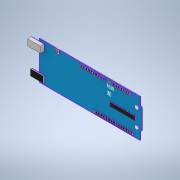
# Autodesk Inventor part: Arduino board
Saved by Autodesk Inventor 2021 (Build 250183000, 183)
## iProperties
Created: 2021-06-29
Part Number: Arduino board
Material: Generic
Document SubType Name: Modeling
Designer: shifa
Density: 1 g/cm^3
Appearance: Default
Author: shifa
Autodesk Inventor part; units mm, degrees
ref_plane "YZ Plane" through (0, 0, 0) normal (1, 0, 0) x (0, 1, 0)
ref_plane "XZ Plane" through (0, 0, 0) normal (0, 1, 0) x (-1, 0, 0)
ref_plane "XY Plane" through (0, 0, 0) normal (0, 0, 1) x (1, 0, 0)
sketch "Sketch1" plane through (0, 0, 0) normal (0, 0, 1) x (1, 0, 0)
  line L0 (-70, -14.9942) -> (-70, 15.0058)
  line L1 (-70, 15.0058) -> (10, 15.0058)
  line L2 (10, 15.0058) -> (10, 9)
  line L3 (10, 9) -> (11.2892, 8.1067)
  line L4 (11.2892, 8.1067) -> (11.2892, -7.6953)
  line L5 (11.2892, -7.6953) -> (10, -8.7379)
  line L6 (10, -8.7379) -> (10, -14.9942)
  line L7 (10, -14.9942) -> (-70, -14.9942)
  line L8 (-56.9712, 15.0058) -> (-53.9712, 15.0058)
  line L9 (-53.9712, 15.0058) -> (-53.9712, 12.0058)
  line L10 (-53.9712, 12.0058) -> (-56.9712, 12.0058)
  line L11 (-56.9712, 12.0058) -> (-56.9712, 15.0058)
  circle A0 centre (-55.5993, 13.6025) radius 1
  line L12 (-76.1027, 13.1862) -> (-66.1027, 13.1862)
  line L13 (-66.1027, 13.1862) -> (-66.1027, 8.1862)
  line L14 (-66.1027, 8.1862) -> (-76.1027, 8.1862)
  line L15 (-76.1027, 8.1862) -> (-76.1027, 13.1862)
  line L16 (-13.5947, -0.1189) -> (6.4053, -0.1189)
  line L17 (6.4053, -0.1189) -> (6.4053, -3.1189)
  line L18 (6.4053, -3.1189) -> (-13.5947, -3.1189)
  line L19 (-13.5947, -3.1189) -> (-13.5947, -0.1189)
  line L20 (-75.8788, -8.319) -> (-65.8788, -8.319)
  line L21 (-65.8788, -8.319) -> (-65.8788, -13.319)
  line L22 (-65.8788, -13.319) -> (-75.8788, -13.319)
  line L23 (-75.8788, -13.319) -> (-75.8788, -8.319)
  circle A1 centre (7.656, 6.6067) radius 1.5
  circle A2 centre (7.656, -7.1392) radius 1.5
  line L24 (2.5046, 14.0058) -> (2.5046, 12.0058)
  line L25 (2.5046, 12.0058) -> (-14.4954, 12.0058)
  line L26 (-14.4954, 14.0058) -> (2.5046, 14.0058)
  line L27 (-14.4954, 12.0058) -> (-14.4954, 14.0058)
  line L28 (-17.3599, 14.0058) -> (-17.3599, 12.0058)
  line L29 (-17.3599, 12.0058) -> (-37.8599, 12.0058)
  line L30 (-37.8599, 14.0058) -> (-17.3599, 14.0058)
  line L31 (-37.8599, 12.0058) -> (-37.8599, 14.0058)
  line L32 (-14.4954, 14.0058) -> (2.5046, 14.0058)
  line L33 (-14.4954, 12.0058) -> (-14.4954, 14.0058)
  line L34 (2.5046, 12.0058) -> (-14.4954, 12.0058)
  line L35 (2.5046, 14.0058) -> (2.5046, 12.0058)
  line L36 (-8.0961, -12.0647) -> (4.4039, -12.0647)
  line L37 (-8.0961, -14.0647) -> (-8.0961, -12.0647)
  line L38 (4.4039, -14.0647) -> (-8.0961, -14.0647)
  line L39 (4.4039, -12.0647) -> (4.4039, -14.0647)
  line L40 (-26.6201, -12.0647) -> (-9.6201, -12.0647)
  line L41 (-26.6201, -14.0647) -> (-26.6201, -12.0647)
  line L42 (-9.6201, -14.0647) -> (-26.6201, -14.0647)
  line L43 (-9.6201, -12.0647) -> (-9.6201, -14.0647)
  line L44 (-37.2773, 13.7542) -> (-35.7773, 13.7542)
  line L45 (-35.7773, 13.7542) -> (-35.7773, 12.2542)
  line L46 (-35.7773, 12.2542) -> (-37.2773, 12.2542)
  line L47 (-37.2773, 12.2542) -> (-37.2773, 13.7542)
  line L48 (-35.2773, 13.7542) -> (-33.7773, 13.7542)
  line L49 (-35.2773, 12.2542) -> (-35.2773, 13.7542)
  line L50 (-33.7773, 12.2542) -> (-35.2773, 12.2542)
  line L51 (-33.7773, 13.7542) -> (-33.7773, 12.2542)
  line L52 (-33.2773, 13.7542) -> (-31.7773, 13.7542)
  line L53 (-33.2773, 12.2542) -> (-33.2773, 13.7542)
  line L54 (-31.7773, 12.2542) -> (-33.2773, 12.2542)
  line L55 (-31.7773, 13.7542) -> (-31.7773, 12.2542)
  line L56 (-31.2773, 13.7542) -> (-29.7773, 13.7542)
  line L57 (-31.2773, 12.2542) -> (-31.2773, 13.7542)
  line L58 (-29.7773, 12.2542) -> (-31.2773, 12.2542)
  line L59 (-29.7773, 13.7542) -> (-29.7773, 12.2542)
  line L60 (-29.2773, 13.7542) -> (-27.7773, 13.7542)
  line L61 (-29.2773, 12.2542) -> (-29.2773, 13.7542)
  line L62 (-27.7773, 12.2542) -> (-29.2773, 12.2542)
  line L63 (-27.7773, 13.7542) -> (-27.7773, 12.2542)
  line L64 (-27.2773, 13.7542) -> (-25.7773, 13.7542)
  line L65 (-27.2773, 12.2542) -> (-27.2773, 13.7542)
  line L66 (-25.7773, 12.2542) -> (-27.2773, 12.2542)
  line L67 (-25.7773, 13.7542) -> (-25.7773, 12.2542)
  line L68 (-25.2773, 13.7542) -> (-23.7773, 13.7542)
  line L69 (-25.2773, 12.2542) -> (-25.2773, 13.7542)
  line L70 (-23.7773, 12.2542) -> (-25.2773, 12.2542)
  line L71 (-23.7773, 13.7542) -> (-23.7773, 12.2542)
  line L72 (-23.2773, 13.7542) -> (-21.7773, 13.7542)
  line L73 (-23.2773, 12.2542) -> (-23.2773, 13.7542)
  line L74 (-21.7773, 12.2542) -> (-23.2773, 12.2542)
  line L75 (-21.7773, 13.7542) -> (-21.7773, 12.2542)
  line L76 (-21.2773, 13.7542) -> (-19.7773, 13.7542)
  line L77 (-21.2773, 12.2542) -> (-21.2773, 13.7542)
  line L78 (-19.7773, 12.2542) -> (-21.2773, 12.2542)
  line L79 (-19.7773, 13.7542) -> (-19.7773, 12.2542)
  line L80 (-19.2773, 13.7542) -> (-17.7773, 13.7542)
  line L81 (-19.2773, 12.2542) -> (-19.2773, 13.7542)
  line L82 (-17.7773, 12.2542) -> (-19.2773, 12.2542)
  line L83 (-17.7773, 13.7542) -> (-17.7773, 12.2542)
  line L84 (-25.4265, -12.3263) -> (-23.9265, -12.3263)
  line L85 (-23.9265, -12.3263) -> (-23.9265, -13.8263)
  line L86 (-23.9265, -13.8263) -> (-25.4265, -13.8263)
  line L87 (-25.4265, -13.8263) -> (-25.4265, -12.3263)
  line L88 (-13.5947, 13.7542) -> (-12.0947, 13.7542)
  line L89 (-12.0947, 13.7542) -> (-12.0947, 12.2542)
  line L90 (-12.0947, 12.2542) -> (-13.5947, 12.2542)
  line L91 (-13.5947, 12.2542) -> (-13.5947, 13.7542)
  line L92 (-7.6221, -12.359) -> (-6.1221, -12.359)
  line L93 (-6.1221, -12.359) -> (-6.1221, -13.859)
  line L94 (-6.1221, -13.859) -> (-7.6221, -13.859)
  line L95 (-7.6221, -13.859) -> (-7.6221, -12.359)
  line L96 (-11.5947, 13.7542) -> (-10.0947, 13.7542)
  line L97 (-11.5947, 12.2542) -> (-11.5947, 13.7542)
  line L98 (-10.0947, 13.7542) -> (-10.0947, 12.2542)
  line L99 (-10.0947, 12.2542) -> (-11.5947, 12.2542)
  line L100 (-9.5947, 13.7542) -> (-8.0947, 13.7542)
  line L101 (-9.5947, 12.2542) -> (-9.5947, 13.7542)
  line L102 (-8.0947, 13.7542) -> (-8.0947, 12.2542)
  line L103 (-8.0947, 12.2542) -> (-9.5947, 12.2542)
  line L104 (-7.5947, 13.7542) -> (-6.0947, 13.7542)
  line L105 (-7.5947, 12.2542) -> (-7.5947, 13.7542)
  line L106 (-6.0947, 13.7542) -> (-6.0947, 12.2542)
  line L107 (-6.0947, 12.2542) -> (-7.5947, 12.2542)
  line L108 (-5.5947, 13.7542) -> (-4.0947, 13.7542)
  line L109 (-5.5947, 12.2542) -> (-5.5947, 13.7542)
  line L110 (-4.0947, 13.7542) -> (-4.0947, 12.2542)
  line L111 (-4.0947, 12.2542) -> (-5.5947, 12.2542)
  line L112 (-3.5947, 13.7542) -> (-2.0947, 13.7542)
  line L113 (-3.5947, 12.2542) -> (-3.5947, 13.7542)
  line L114 (-2.0947, 13.7542) -> (-2.0947, 12.2542)
  line L115 (-2.0947, 12.2542) -> (-3.5947, 12.2542)
  line L116 (-1.5947, 13.7542) -> (-0.0947, 13.7542)
  line L117 (-1.5947, 12.2542) -> (-1.5947, 13.7542)
  line L118 (-0.0947, 13.7542) -> (-0.0947, 12.2542)
  line L119 (-0.0947, 12.2542) -> (-1.5947, 12.2542)
  line L120 (0.4053, 13.7542) -> (1.9053, 13.7542)
  line L121 (0.4053, 12.2542) -> (0.4053, 13.7542)
  line L122 (1.9053, 13.7542) -> (1.9053, 12.2542)
  line L123 (1.9053, 12.2542) -> (0.4053, 12.2542)
  line L124 (-23.4265, -12.3263) -> (-21.9265, -12.3263)
  line L125 (-23.4265, -13.8263) -> (-23.4265, -12.3263)
  line L126 (-21.9265, -12.3263) -> (-21.9265, -13.8263)
  line L127 (-21.9265, -13.8263) -> (-23.4265, -13.8263)
  line L128 (-21.4265, -12.3263) -> (-19.9265, -12.3263)
  line L129 (-21.4265, -13.8263) -> (-21.4265, -12.3263)
  line L130 (-19.9265, -12.3263) -> (-19.9265, -13.8263)
  line L131 (-19.9265, -13.8263) -> (-21.4265, -13.8263)
  line L132 (-19.4265, -12.3263) -> (-17.9265, -12.3263)
  line L133 (-19.4265, -13.8263) -> (-19.4265, -12.3263)
  line L134 (-17.9265, -12.3263) -> (-17.9265, -13.8263)
  line L135 (-17.9265, -13.8263) -> (-19.4265, -13.8263)
  line L136 (-17.4265, -12.3263) -> (-15.9265, -12.3263)
  line L137 (-17.4265, -13.8263) -> (-17.4265, -12.3263)
  line L138 (-15.9265, -12.3263) -> (-15.9265, -13.8263)
  line L139 (-15.9265, -13.8263) -> (-17.4265, -13.8263)
  line L140 (-15.4265, -12.3263) -> (-13.9265, -12.3263)
  line L141 (-15.4265, -13.8263) -> (-15.4265, -12.3263)
  line L142 (-13.9265, -12.3263) -> (-13.9265, -13.8263)
  line L143 (-13.9265, -13.8263) -> (-15.4265, -13.8263)
  line L144 (-13.4265, -12.3263) -> (-11.9265, -12.3263)
  line L145 (-13.4265, -13.8263) -> (-13.4265, -12.3263)
  line L146 (-11.9265, -12.3263) -> (-11.9265, -13.8263)
  line L147 (-11.9265, -13.8263) -> (-13.4265, -13.8263)
  line L148 (-11.4265, -12.3263) -> (-9.9265, -12.3263)
  line L149 (-11.4265, -13.8263) -> (-11.4265, -12.3263)
  line L150 (-9.9265, -12.3263) -> (-9.9265, -13.8263)
  line L151 (-9.9265, -13.8263) -> (-11.4265, -13.8263)
  line L152 (-5.6221, -12.359) -> (-4.1221, -12.359)
  line L153 (-5.6221, -13.859) -> (-5.6221, -12.359)
  line L154 (-4.1221, -12.359) -> (-4.1221, -13.859)
  line L155 (-4.1221, -13.859) -> (-5.6221, -13.859)
  line L156 (-3.6221, -12.359) -> (-2.1221, -12.359)
  line L157 (-3.6221, -13.859) -> (-3.6221, -12.359)
  line L158 (-2.1221, -12.359) -> (-2.1221, -13.859)
  line L159 (-2.1221, -13.859) -> (-3.6221, -13.859)
  line L160 (-1.6221, -12.359) -> (-0.1221, -12.359)
  line L161 (-1.6221, -13.859) -> (-1.6221, -12.359)
  line L162 (-0.1221, -12.359) -> (-0.1221, -13.859)
  line L163 (-0.1221, -13.859) -> (-1.6221, -13.859)
  line L164 (0.3779, -12.359) -> (1.8779, -12.359)
  line L165 (0.3779, -13.859) -> (0.3779, -12.359)
  line L166 (1.8779, -12.359) -> (1.8779, -13.859)
  line L167 (1.8779, -13.859) -> (0.3779, -13.859)
  line L168 (2.3779, -12.359) -> (3.8779, -12.359)
  line L169 (2.3779, -13.859) -> (2.3779, -12.359)
  line L170 (3.8779, -12.359) -> (3.8779, -13.859)
  line L171 (3.8779, -13.859) -> (2.3779, -13.859)
  point P0 (-70, 13.1862)
  point P1 (-70, 8.1862)
  point P2 (-70, -8.319)
  point P3 (-70, -13.319)
  dimension "d53" = 1
  dimension "d54" = 10
  dimension "d0" = 30
  dimension "d1" = 80
  dimension "d87" = 3
  dimension "d88" = 3
  dimension "d107" = 10
  dimension "d108" = 5
  dimension "d109" = 10
  dimension "d110" = 5
  dimension "d113" = 20
  dimension "d114" = 3
  dimension "d115" = 3
  dimension "d116" = 3
  dimension "d117" = 2
  dimension "d122" = 17
  dimension "d123" = 2
  dimension "d124" = 20.5
  dimension "d125" = 2
  dimension "d126" = 17
  dimension "d127" = 2
  dimension "d128" = 12.5
  dimension "d129" = 2
  dimension "d130" = 17
  dimension "d131" = 2
  dimension "d132" = 1.5
  dimension "d133" = 1.5
  dimension "d136" = 2
  dimension "d145" = 1.5
  dimension "d146" = 1.5
  dimension "d151" = 1.5
  dimension "d152" = 1.5
  dimension "d157" = 1.5
  dimension "d158" = 1.5
  dimension "d161" = 2
  dimension "d168" = 2
  dimension "d175" = 2
  constraints: 344 end point, 8 horizontal, 8 parallel, 4 perpendicular, 3 centre point, 3 point on line, 224 other
  measures "d0" distance of L0.start L0.end
  measures "d1" distance of L0.end L1.end
  measures "d87" diameter of A1
  measures "d88" diameter of A2
  measures "d107" distance of L12.start L12.end
  measures "d108" distance of L12.end L13.end
  measures "d109" distance of L20.start L20.end
  measures "d110" distance of L20.end L21.end
  measures "d113" distance of L16.start L16.end
  measures "d114" distance of L18.end L16.start
  measures "d115" distance of L9.end L10.end
  measures "d116" distance of L10.end L8.start
  measures "d117" diameter of A0
  measures "d122" distance of L26.start L26.end
  measures "d123" distance of L27.start L26.start
  measures "d124" distance of L30.start L30.end
  measures "d125" distance of L31.start L30.start
  measures "d126" distance of L33.end L32.end
  measures "d127" distance of L33.start L33.end
  measures "d128" distance of L37.end L36.end
  measures "d129" distance of L37.start L37.end
  measures "d130" distance of L41.end L40.end
  measures "d131" distance of L41.start L41.end
  measures "d132" distance of L45.end L46.end
  measures "d133" distance of L44.end L45.end
  measures "d136" distance of L44.start L48.start
  measures "d145" distance of L85.end L87.start
  measures "d146" distance of L84.end L85.end
  measures "d151" distance of L89.end L91.start
  measures "d152" distance of L88.end L89.end
  measures "d157" distance of L93.end L95.start
  measures "d158" distance of L92.end L93.end
  measures "d161" distance of L88.start L96.start
  measures "d168" distance of L84.start L124.start
  measures "d175" distance of L92.start L152.start
extrude "Extrusion1" add sketch "Sketch1" along normal blind 3 contours L14 L15 L12 L0 | L0 L12 L13 L14
extrude "Extrusion2" add sketch "Sketch1" along normal blind 1 contours L22 L23 L20 L0 | L0 L20 L21 L22
extrude "Extrusion3" add sketch "Sketch1" along normal blind 0.5 contours L16 L17 L18 L19
extrude "Extrusion4" add sketch "Sketch1" against normal blind 0.5 contours L0 L22 L21 L20 L14 L13 L12 L1 L11 L10 L9 L2 L3 L4 L5 L6 L7 | L24 L25 L27 L26 | L28 L29 L31 L30 | L36 L39 L38 L37 | L40 L43 L42 L41 | L44 L45 L46 L47 | L48 L51 L50 L49 | L52 L55 L54 L53 | L56 L59 L58 L57 | L60 L63 L62 L61 | L64 L67 L66 L65 | L68 L71 L70 L69 | L72 L75 L74 L73 | L76 L79 L78 L77 | L80 L83 L82 L81 | L84 L85 L86 L87 | L88 L89 L90 L91 | L92 L93 L94 L95 | L96 L98 L99 L97 | L100 L102 L103 L101 | L104 L106 L107 L105 | L108 L110 L111 L109 | L112 L114 L115 L113 | L116 L118 L119 L117 | L120 L122 L123 L121 | L124 L126 L127 L125 | L128 L130 L131 L129 | L132 L134 L135 L133 | L136 L138 L139 L137 | L140 L142 L143 L141 | L144 L146 L147 L145 | L148 L150 L151 L149 | L152 L154 L155 L153 | L156 L158 L159 L157 | L160 L162 L163 L161 | L164 L166 L167 L165 | L168 L170 L171 L169
extrude "Extrusion8" add sketch "Sketch1" along normal blind 0.2 contours L1 L9 L10 L11
extrude "Extrusion9" add sketch "Sketch1" along normal blind 0.5 contours A0 | A1 | A2
sketch "Sketch2" plane through (0, 0, 0) normal (0, 0, 1) x (1, 0, 0)
  point P0 (0, 0)
sketch "Sketch3" plane through (0, 0, 0) normal (0, 0, 1) x (1, 0, 0)
  point P0 (0, 0)
sketch "Sketch4" plane through (0, 0, 0) normal (0, 1, 0) x (-1, 0, 0)
  point P0 (0, 0)
  point P1 (0, 0)
  constraints: 1 coincident
sketch "Sketch5" plane through (0, 0, 0) normal (0, 0, 1) x (1, 0, 0)
  point P0 (0, 0)
sketch "Sketch6" plane through (0, 0, 0) normal (0, 0, 1) x (1, 0, 0)
  line L0 (-16.3152, 11.5204) -> (-9.3, 11.5204) construction
  line L1 (-9.3, 11.5204) -> (-9.3, 9.9114) construction
  line L2 (-9.3, 9.9114) -> (-16.3152, 9.9114) construction
  line L3 (-16.3152, 9.9114) -> (-16.3152, 11.5204) construction
  point P0 (0, 0)
  constraints: 2 other
sketch "Sketch7" plane through (0, 0, 0) normal (0, 0, 1) x (1, 0, 0)
  point P0 (0, 0)
sketch "Sketch8" plane through (0, 0, 0) normal (0, 0, 1) x (1, 0, 0)
  point P0 (0, 0)
extrude "Extrusion10" cut sketch "Sketch1" against normal blind 0.1 contours L44 L45 L46 L47 | L48 L51 L50 L49 | L52 L55 L54 L53 | L56 L59 L58 L57 | L60 L63 L62 L61 | L64 L67 L66 L65 | L68 L71 L70 L69 | L72 L75 L74 L73 | L76 L79 L78 L77 | L80 L83 L82 L81 | L84 L85 L86 L87 | L88 L89 L90 L91 | L92 L93 L94 L95 | L96 L98 L99 L97 | L100 L102 L103 L101 | L104 L106 L107 L105 | L108 L110 L111 L109 | L112 L114 L115 L113 | L116 L118 L119 L117 | L120 L122 L123 L121 | L124 L126 L127 L125 | L128 L130 L131 L129 | L132 L134 L135 L133 | L136 L138 L139 L137 | L140 L142 L143 L141 | L144 L146 L147 L145 | L148 L150 L151 L149 | L152 L154 L155 L153 | L156 L158 L159 L157 | L160 L162 L163 L161 | L164 L166 L167 L165 | L168 L170 L171 L169
extrude "Extrusion11" add sketch "Sketch1" along normal blind 0.5 contours L24 L25 L27 L26 | L28 L29 L31 L30 | L36 L39 L38 L37 | L40 L43 L42 L41
body "Solid1"
